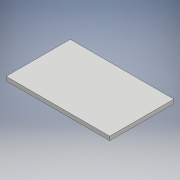
# Autodesk Inventor part: Eletronica - suporteArduino
Saved by Autodesk Inventor 2017 (Build 210142000, 142)
## iProperties
Created: 2020-10-10
Part Number: Eletronica - suporteArduino
Material: Generic
Document SubType Name: Modeling
Designer: ale
Density: 1 g/cm^3
Appearance: Default
Author: ale
Autodesk Inventor part; units mm, degrees
ref_plane "YZ Plane" through (0, 0, 0) normal (1, 0, 0) x (0, 1, 0)
ref_plane "XZ Plane" through (0, 0, 0) normal (0, 1, 0) x (-1, 0, 0)
ref_plane "XY Plane" through (0, 0, 0) normal (0, 0, 1) x (1, 0, 0)
sketch "Sketch1" plane through (0, 0, 0) normal (0, 0, 1) x (1, 0, 0)
  line L0 (-52.5, 32.5) -> (52.5, 32.5)
  line L1 (52.5, 32.5) -> (52.5, -32.5)
  line L2 (52.5, -32.5) -> (-52.5, -32.5)
  line L3 (-52.5, -32.5) -> (-52.5, 32.5)
  line L4 (-52.5, 32.5) -> (52.5, -32.5) construction
  line L5 (52.5, 32.5) -> (-52.5, -32.5) construction
  point P0 (0, 0)
  dimension "d0" = 105
  dimension "d1" = 65
  constraints: 12 end point, 2 midpoint, 2 parallel, 1 horizontal, 1 perpendicular
  measures "d0" distance of L1.end L2.end
  measures "d1" distance of L0.end L1.end
extrude "Extrusion1" add sketch "Sketch1" along normal blind 4
body "Solid1"
